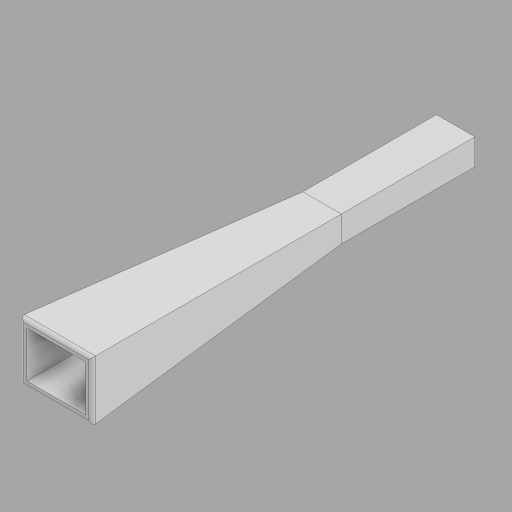
# Autodesk Inventor part: RWG_Horn_ProbeAntennaV1
Saved by Autodesk Inventor 2023 (Build 270158000, 158)
## iProperties
Created: 2024-09-19
Part Number: RWG_Horn_ProbeAntennaV1
Material: Generisch
Document SubType Name: Modeling
Designer: Nils Bade
Density: 1 g/cm^3
Appearance: Vorgabe
Author: Nils Bade
Autodesk Inventor part; units mm, degrees
ref_plane "YZ Plane" through (0, 0, 0) normal (1, 0, 0) x (0, 1, 0)
ref_plane "XZ Plane" through (0, 0, 0) normal (0, 1, 0) x (-1, 0, 0)
sketch "Skizze1" plane through (0, 0, 0) normal (0, 0, 1) x (1, 0, 0)
  line L0 (1.8795, 0.94) -> (-1.8795, 0.94)
  line L1 (-1.8795, 0.94) -> (-1.8795, -0.94)
  line L2 (-1.8795, -0.94) -> (1.8795, -0.94)
  line L3 (1.8795, -0.94) -> (1.8795, 0.94)
  line L4 (1.8795, 0.94) -> (-1.8795, -0.94) construction
  line L5 (-1.8795, 0.94) -> (1.8795, -0.94) construction
  line L6 (-2.8795, -1.94) -> (-2.8795, 1.94)
  line L7 (-2.8795, 1.94) -> (2.8795, 1.94)
  line L8 (2.8795, 1.94) -> (2.8795, -1.94)
  line L9 (2.8795, -1.94) -> (-2.8795, -1.94)
  point P0 (0, 0)
  dimension "d0" = 1.88
  dimension "d1" = 3.759
  dimension "d2" = 1
  constraints: 20 end point, 4 parallel, 2 midpoint, 2 perpendicular, 1 horizontal, 3 other
  measures "d0" distance between parallel lines of L2 L0
  measures "d1" distance between parallel lines of L3 L1
  measures "d2" distance between parallel lines of L1 L6
extrude "Ex1-RWG" add sketch "Skizze1" along normal blind 20
ref_plane "Endebene" through (0, 0, 59.75) normal (0, 0, 1) x (1, 0, 0)
sketch "S-Hornöffnung" plane through (0, 0, 59.75) normal (0, 0, 1) x (1, 0, 0)
  line L0 (2.8795, -1.94) -> (2.8795, 1.94) projected
  line L1 (2.8795, 1.94) -> (-2.8795, 1.94) projected
  line L2 (-2.8795, 1.94) -> (-2.8795, -1.94) projected
  line L3 (-2.8795, -1.94) -> (2.8795, -1.94) projected
  line L4 (1.8795, 0.94) -> (1.8795, -0.94) projected
  line L5 (1.8795, -0.94) -> (-1.8795, -0.94) projected
  line L6 (-1.8795, -0.94) -> (-1.8795, 0.94) projected
  line L7 (-1.8795, 0.94) -> (1.8795, 0.94) projected
  line L8 (4.3795, 3.44) -> (4.3795, -3.44)
  line L9 (4.3795, -3.44) -> (-4.3795, -3.44)
  line L10 (-4.3795, -3.44) -> (-4.3795, 3.44)
  line L11 (-4.3795, 3.44) -> (4.3795, 3.44)
  line L12 (5.3795, -4.44) -> (5.3795, 4.44)
  line L13 (5.3795, 4.44) -> (-5.3795, 4.44)
  line L14 (-5.3795, 4.44) -> (-5.3795, -4.44)
  line L15 (-5.3795, -4.44) -> (5.3795, -4.44)
  point P0 (0, 0)
  dimension "d19" = 2.5
  dimension "d20" = 1
  constraints: 16 end point, 6 other
  measures "d19" distance between parallel lines of L7 L11
  measures "d20" distance between parallel lines of L8 L12
sketch "S-RWGÜbergang" plane through (0, 0, 20) normal (0, 0, 1) x (1, 0, 0)
  line L0 (2.8795, -1.94) -> (2.8795, 1.94) projected
  line L1 (2.8795, 1.94) -> (-2.8795, 1.94) projected
  line L2 (-2.8795, 1.94) -> (-2.8795, -1.94) projected
  line L3 (-2.8795, -1.94) -> (2.8795, -1.94) projected
  line L4 (1.8795, 0.94) -> (1.8795, -0.94) projected
  line L5 (1.8795, -0.94) -> (-1.8795, -0.94) projected
  line L6 (-1.8795, -0.94) -> (-1.8795, 0.94) projected
  line L7 (-1.8795, 0.94) -> (1.8795, 0.94) projected
  point P0 (0, 0)
loft "Erhebung-Horn1" add profiles "S-Hornöffnung" section 1 edges at (2.8795, 0, 20) (0, 1.94, 20) (-2.8795, 0, 20) (0, -1.94, 20) contours L3 L2 L1 L0 | L4 L5 L6 L7 | L8 L9 L10 L11 | L15 L14 L13 L12
loft "Erhebung-Horn2" cut profiles "S-Hornöffnung" section 1 edges at (0, 0.94, 20) (1.8795, 0, 20) (0, -0.94, 20) (-1.8795, 0, 20) contours L3 L2 L1 L0 | L4 L5 L6 L7 | L8 L9 L10 L11
fillet "Rundung-0.5mm" radius 0.5 4 edges at (0, 4.44, 59.75) (-5.3795, 0, 59.75) (0, -4.44, 59.75) (5.3795, 0, 59.75)
fillet_without_effect "Rundung-10mm"
